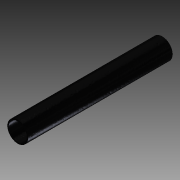
# Autodesk Inventor part: Sleeve
Saved by Autodesk Inventor 2013 (Build 170138000, 138)
## iProperties
Created: 2014-05-23
Part Number: Sleeve
Material: Rubber
Document SubType Name: Modeling
Designer: ryclifton
Density: 0.93 g/cm^3
Mass: 30.8812 g
Surface Area: 351.883 cm^2
Volume: 33.2056 cm^3
Author: ryclifton
Autodesk Inventor part; units mm, degrees
ref_plane "YZ Plane" through (0, 0, 0) normal (1, 0, 0) x (0, 1, 0)
ref_plane "XZ Plane" through (0, 0, 0) normal (0, 1, 0) x (-1, 0, 0)
ref_plane "XY Plane" through (0, 0, 0) normal (0, 0, 1) x (1, 0, 0)
sketch "Sketch1" plane through (0, 0, 0) normal (0, 0, 1) x (1, 0, 0)
  circle A0 centre (0, 0) radius 14.605
  dimension "d0" = 29.21
  constraints: 1 centre point, 1 coincident
  measures "d0" diameter of A0
extrude "Extrusion1" add sketch "Sketch1" along normal blind 203.2
sketch "Sketch3" plane through (0, 0, 203.2) normal (0, 0, 1) x (1, 0, 0)
  circle A0 centre (0, 0) radius 14.605 projected
  circle A1 centre (0, 0) radius 12.7
  dimension "d10" = 25.4
  constraints: 1 centre point, 1 coincident
  measures "d10" diameter of A1
extrude "Extrusion3" cut sketch "Sketch3" against normal blind 203.2 contours A1
body "Solid1"
